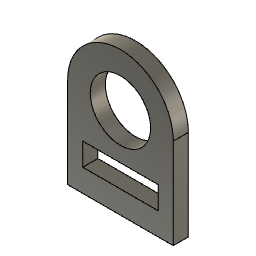
Exercise_01 (Autodesk Fusion 360 design; units mm, degrees)
Autodesk Fusion 360 part; units mm, degrees
sketch "Sketch1" plane through (0, 0, 0) normal (0, 1, 0) x (1, 0, 0)
  line L0 (35, 0) -> (-35, 0)
  line L1 (-35, 0) -> (-35, -60)
  line L2 (-35, -60) -> (35, -60)
  line L3 (35, -60) -> (35, 0)
  line L4 (35, 0) -> (-35, -60) construction
  line L5 (-35, 0) -> (35, -60) construction
  line L6 (-35, -60) -> (35, -60) construction
  circle A0 centre (0, -60) radius 35
  circle A1 centre (0, -60) radius 20
  line L7 (0, 0) -> (0, -15) construction
  line L8 (-35, -15) -> (-25, -15) construction
  line L9 (-25, -15) -> (25, -15)
  line L10 (25, -15) -> (25, -30)
  line L11 (25, -30) -> (-25, -30)
  line L12 (-25, -30) -> (-25, -15)
  point P0 (0, -30)
  dimension "d1" = 70
  dimension "d2" = 70
  dimension "d3" = 40
  dimension "d4" = 15
  dimension "d5" = 10
  dimension "d6" = 50
  dimension "d7" = 15
  constraint horizontal L0
  constraint perpendicular L0 L1
  constraint parallel L0 L2
  constraint parallel L1 L3
  constraint coincident L4 P0
  constraint coincident L5 P0
  constraint midpoint L6 A0.centre
  constraint concentric A0 A1
  constraint coincident L7.start origin
  constraint perpendicular L0 L7
  constraint coincident L1 L8.start
  constraint perpendicular L1 L8
  constraint horizontal L9
  constraint vertical L10
  constraint horizontal L11
  constraint vertical L12
  measures "d1" distance of L1.end L2.end
  measures "d2" diameter of A0
  measures "d3" diameter of A1
  measures "d4" distance of L7.start L7.end
  measures "d5" distance of L8.start L8.end
  measures "d6" distance of L8.end L9.end
  measures "d7" distance of L8.end L11.end
extrude "Extrude1" add sketch "Sketch1" along normal mid plane 10 contours L0 L1 L3 A0 L9 L10 L11 L12 | L2 A0 A1 | L2 A0 A1 L11 | A0 L11 | A0 L9 L10 L11 L12
extrude "Extrude2" cut sketch "Sketch1" along normal mid plane 60 contours A0 L11 | A0 L9 L10 L11 L12
